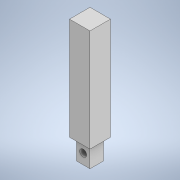
# Autodesk Inventor part: Pendulum
Saved by Autodesk Inventor 2021 (Build 250183000, 183)
## iProperties
Created: 2022-10-04
Part Number: Pendulum
Material: Generic
Document SubType Name: Modeling
Designer: mrizw
Density: 1 g/cm^3
Appearance: Default
Author: mrizw
Autodesk Inventor part; units mm, degrees
ref_plane "YZ Plane" through (0, 0, 0) normal (1, 0, 0) x (0, 1, 0)
ref_plane "XZ Plane" through (0, 0, 0) normal (0, 1, 0) x (-1, 0, 0)
ref_plane "XY Plane" through (0, 0, 0) normal (0, 0, 1) x (1, 0, 0)
sketch "Sketch1" plane through (0, 0, 0) normal (0, 1, 0) x (-1, 0, 0)
  line L0 (0, 0) -> (-10, 0)
  line L1 (-10, 0) -> (-10, -10)
  line L2 (-10, -10) -> (0, -10)
  line L3 (0, -10) -> (0, 0)
  dimension "d0" = 10
  dimension "d1" = 10
  constraints: 8 end point, 2 parallel, 1 horizontal, 1 perpendicular
  measures "d0" distance of L2.end L1.end
  measures "d1" distance of L1.end L0.end
extrude "Extrusion1" add sketch "Sketch1" along normal blind 15
sketch "Sketch2" plane through (0, 15, 0) normal (0, 1, 0) x (1, 0, 0)
  line L0 (12.5, -2.5) -> (-2.5, -2.5)
  line L1 (-2.5, -2.5) -> (-2.5, 12.5)
  line L2 (-2.5, 12.5) -> (12.5, 12.5)
  line L3 (12.5, 12.5) -> (12.5, -2.5)
  line L4 (12.5, -2.5) -> (-2.5, 12.5) construction
  line L5 (-2.5, -2.5) -> (12.5, 12.5) construction
  point P0 (0, 0)
  point P1 (5, 5)
  dimension "d4" = 15
  dimension "d5" = 15
  constraints: 12 end point, 2 midpoint, 2 parallel, 1 horizontal, 1 perpendicular
  measures "d4" distance of L1.end L2.end
  measures "d5" distance of L0.end L1.end
extrude "Extrusion2" add sketch "Sketch2" along normal blind 75
sketch "Sketch3" plane through (0, 0, 0) normal (0, 0, 1) x (1, 0, 0)
  line L0 (0, 0) -> (0, 15) projected
  line L1 (0, 7.5) -> (10, 7.5)
  line L2 (10, 0) -> (10, 15) projected
  line L3 (-2.5, 15) -> (12.5, 15) projected
  line L4 (5, 15) -> (5, 0)
  line L5 (0, 0) -> (10, 0) projected
  point P0 (5, 7.5)
  constraints: 5 midpoint, 4 end point
hole "Hole1" at (5, 7.5, 0) direction (0, 0, -1) diameter 5 end through all
body "Solid1"
